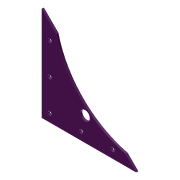
# Autodesk Inventor part: CylinderOffsetPlate
Saved by Autodesk Inventor 2012 (Build 160160000, 160)
## iProperties
Created: 2013-01-19
Part Number: CylinderOffsetPlate
Material: Aluminum-6061
Document SubType Name: Modeling
Designer: JesseK
Density: 2.71 g/cm^3
Mass: 76.387 g
Surface Area: 199.086 cm^2
Volume: 28.1871 cm^3
Author: JesseK
Autodesk Inventor part; units mm, degrees
ref_plane "YZ Plane" through (0, 0, 0) normal (1, 0, 0) x (0, 1, 0)
ref_plane "XZ Plane" through (0, 0, 0) normal (0, 1, 0) x (-1, 0, 0)
ref_plane "XY Plane" through (0, 0, 0) normal (0, 0, 1) x (1, 0, 0)
sketch "Sketch1" plane through (0, 0, 0) normal (0, 0, 1) x (1, 0, 0)
  circle A0 centre (79.9619, 51.3388) radius 7.9375
  line L0 (10.1119, 165.6388) -> (10.1119, 13.2388)
  line L1 (10.1119, 13.2388) -> (162.5119, 13.2388)
  line L2 (162.5119, 13.2388) -> (10.1119, 165.6388)
  point P0 (0, 0)
  dimension "d0" = 15.875
  dimension "d1" = 152.4
  dimension "d2" = 152.4
  dimension "d3" = 38.1
  dimension "d4" = 69.85
  constraints: 6 end point, 1 centre point, 1 horizontal, 1 vertical
  measures "d0" diameter of A0
  measures "d1" distance of L0.start L0.end
  measures "d2" distance of L0.end L1.end
  measures "d3" distance from line of L1 A0.centre
  measures "d4" distance from line of L0 A0.centre
extrude "Extrusion1" add sketch "Sketch1" along normal blind 3.175
sketch "Sketch2" plane through (0, 0, 3.175) normal (0, 0, 1) x (1, 0, 0)
  line L0 (10.1119, 13.2388) -> (10.1119, 165.6388) projected
  line L1 (162.5119, 13.2388) -> (10.1119, 13.2388) projected
  circle A0 centre (22.8119, 76.7388) radius 3.175
  circle A1 centre (73.6119, 25.9388) radius 3.175
  circle A2 centre (22.8119, 25.9388) radius 3.175
  line L2 (22.8119, 76.7388) -> (22.8119, 25.9388) construction
  line L3 (22.8119, 25.9388) -> (73.6119, 25.9388) construction
  point P0 (0, 0)
  dimension "d7" = 6.35
  dimension "d8" = 12.7
  dimension "d9" = 12.7
  dimension "d10" = 50.8
  dimension "d13" = 50.8
  constraints: 4 end point, 3 centre point, 2 equal radius, 1 horizontal, 1 vertical
  measures "d7" diameter of A1
  measures "d8" distance between parallel lines of L1 L3
  measures "d9" distance between parallel lines of L0 L2
  measures "d10" distance of L2.end L3.end
  measures "d13" distance of L2.start L2.end
extrude "Extrusion2" cut sketch "Sketch2" against normal through all
sketch "Sketch3" plane through (0, 0, 3.175) normal (0, 0, 1) x (1, 0, 0)
  circle A0 centre (22.8119, 25.9388) radius 3.175 projected
  circle A1 centre (22.8119, 127.5388) radius 3.175
  circle A2 centre (124.4119, 25.9388) radius 3.175
  line L0 (22.8119, 127.5388) -> (22.8119, 25.9388) construction
  line L1 (22.8119, 25.9388) -> (124.4119, 25.9388) construction
  point P0 (0, 0)
  dimension "d14" = 6.35
  dimension "d15" = 101.6
  constraints: 4 end point, 2 centre point, 1 equal radius, 1 horizontal, 1 perpendicular, 1 vertical
  measures "d14" diameter of A1
  measures "d15" distance of L0.start L0.end
extrude "Extrusion3" cut sketch "Sketch3" against normal through all contours A1 | A2
sketch "Sketch5" plane through (0, 0, 3.175) normal (0, 0, 1) x (1, 0, 0)
  line L0 (10.1119, 165.6388) -> (162.5119, 13.2388) projected
  arc A0 (33.4951, 142.2556) -> (145.4786, 30.2721) centre (181.5619, 178.3388) ccw
  line L1 (33.4951, 142.2556) -> (145.4786, 30.2721)
  line L2 (10.1119, 13.2388) -> (10.1119, 165.6388) projected
  point P0 (0, 0)
  dimension "d18" = 152.4
  dimension "d25" = 165.1
  dimension "d26" = 171.45
  constraints: 2 end point, 2 point on circle, 2 point on line, 1 centre point, 1 collinear
  measures "d18" radius of A0
  measures "d25" vertical distance of L0.end A0.centre
  measures "d26" distance from line of L2 A0.centre
extrude "Extrusion5" cut sketch "Sketch5" against normal through all
body "Solid1"
